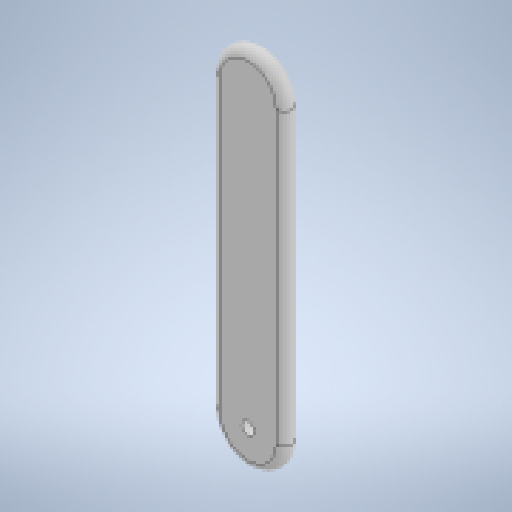
# Autodesk Inventor part: шатун22
Saved by Autodesk Inventor 2023.1 (Build 271208000, 208)
## iProperties
Created: 2024-12-17
Part Number: шатун22
Material: Типовые
Document SubType Name: Modeling
Designer: DELL
Density: 1 g/cm^3
Appearance: По умолчанию
Author: DELL
Autodesk Inventor part; units mm, degrees
ref_plane "YZ Plane" through (0, 0, 0) normal (1, 0, 0) x (0, 1, 0)
ref_plane "XZ Plane" through (0, 0, 0) normal (0, 1, 0) x (-1, 0, 0)
ref_plane "XY Plane" through (0, 0, 0) normal (0, 0, 1) x (1, 0, 0)
sketch "Эскиз1" plane through (0, 0, 0) normal (0, 0, 1) x (1, 0, 0)
  circle A0 centre (0, 0) radius 9
  circle A1 centre (0, 0) radius 1.575
  line L0 (0, -9) -> (0, 99) construction
  line L1 (-9, 0) -> (-9, 90)
  line L2 (9, 90) -> (9, 0)
  arc A2 (-9, 0) -> (9, 0) centre (0, 0) ccw
  arc A3 (9, 90) -> (-9, 90) centre (0, 90) ccw
  point P0 (0, 45)
  dimension "d0" = 18
  dimension "d1" = 3.15
  dimension "d5" = 108
  constraints: 8 end point, 6 point on circle, 4 tangent, 3 centre point, 2 coincident, 2 point on line, 1 midpoint, 1 parallel, 1 vertical, 3 other
  measures "d1" diameter of A1
  measures "d5" distance of L0.start L0.end
extrude "Выдавливание1" add sketch "Эскиз1" along normal blind 4
fillet "Сопряжение1" radius 2 8 edges at (0, 99, 0) (-9, 45, 0) (0, -9, 0) (9, 45, 0) (0, -9, 4) (9, 45, 4) (0, 99, 4) (-9, 45, 4)
